Keyboard Support (Autodesk Fusion 360 design; units mm, degrees)
Autodesk Fusion 360 part; units mm, degrees
sketch "Sketch1" plane through (0, 0, 0) normal (0, 0, 1) x (1, 0, 0)
  line L0 (0, 0) -> (280, 0)
  line L1 (280, 0) -> (280, 6)
  line L2 (280, 6) -> (0, 6)
  line L3 (0, 6) -> (0, 0)
  line L4 (280, 6) -> (0, 6)
  line L5 (0, 6) -> (0, 26)
  line L6 (0, 26) -> (280, 26)
  line L7 (280, 26) -> (280, 6)
  line L8 (140, 26) -> (140, 66) construction
  line L9 (140, 66) -> (150, 66)
  line L10 (150, 66) -> (150, 26)
  line L11 (150, 26) -> (140, 26)
  line L12 (140, 26) -> (140, 66)
  line L13 (140, 66) -> (130, 66)
  line L14 (130, 66) -> (130, 26)
  line L15 (130, 26) -> (140, 26)
  line L16 (140, 26) -> (140, 66)
  dimension "d1" = 280
  dimension "d2" = 6
  dimension "d9" = 20
  dimension "d10" = 280
  dimension "d11" = 40
  dimension "d12" = 10
  dimension "d13" = 10
  constraint horizontal L0
  constraint vertical L1
  constraint horizontal L2
  constraint vertical L3
  constraint coincident L0.start L3.end
  constraint horizontal L4
  constraint vertical L5
  constraint horizontal L6
  constraint vertical L7
  constraint midpoint L6 L8.start
  constraint perpendicular L6 L8
  constraint horizontal L9
  constraint vertical L10
  constraint horizontal L11
  constraint vertical L12
  constraint horizontal L13
  constraint vertical L14
  constraint horizontal L15
  constraint vertical L16
  measures "d1" distance of L0.start L0.end
  measures "d2" distance of L0.start L2.end
  measures "d9" distance of L1.end L6.end
  measures "d10" distance of L5.end L6.end
  measures "d11" distance of L8.start L8.end
  measures "d12" distance of L8.end L9.end
  measures "d13" distance of L8.end L13.end
extrude "Extrude3" add sketch "Sketch1" along normal blind 4 contours L2 L4 L5 L6 L7 L11 L15 makes body 1
extrude "Extrude1" add sketch "Sketch1" along normal blind 10 separate body contours L0 L1 L2 L3 L4 makes body 2
extrude "Extrude4" add sketch "Sketch1" along normal blind 4 contours L6 L12 L13 L14 L15 L16 | L6 L9 L10 L11 L12 L16 bodies 1
sketch "Sketch3" plane through (150, 0, 0) normal (1, 0, 0) x (0, 1, 0)
  line L0 (26, 0) -> (66, 0)
  line L1 (66, 0) -> (66, 4)
  line L2 (66, 4) -> (26, 4)
  line L3 (26, 4) -> (26, 0)
  line L4 (6.0067, 5.0364) -> (66, 1.8987)
  constraint coincident L1 L4.end
extrude "Extrude5" cut sketch "Sketch3" against normal blind 20 contours L1 L2 L3 L4 bodies 1
sketch "Sketch4" plane through (0, 0, 0) normal (0, 0, 1) x (1, 0, 0)
  line L0 (0, -45.217) -> (280, -45.217)
  line L1 (280, -45.217) -> (280, -50.217)
  line L2 (280, -50.217) -> (0, -50.217)
  line L3 (0, -50.217) -> (0, -45.217)
  dimension "d20" = 280
  dimension "d21" = 5
  constraint horizontal L0
  constraint vertical L1
  constraint horizontal L2
  constraint vertical L3
  measures "d20" distance of L0.start L0.end
  measures "d21" distance of L0.start L2.end
extrude "Extrude6" add sketch "Sketch4" along normal blind 5 separate body makes body 3
sketch "Sketch5" plane through (280, 0, 0) normal (1, 0, 0) x (0, 1, 0)
  line L0 (-50.217, 0) -> (-45.217, 0)
  line L1 (-45.217, 0) -> (-45.217, 5)
  line L2 (-45.217, 5) -> (-50.217, 5)
  line L3 (-50.217, 5) -> (-50.217, 0)
  line L4 (-45.217, 5) -> (-50.217, 0)
  constraint coincident L1.end L2.start
  constraint coincident L0.start L3.end
extrude "Extrude7" cut sketch "Sketch5" against normal blind 280 contours L2 L3 L4 bodies 3
fillet "Fillet1" radius 10 2 edges at (130, 66, 0.9493) (150, 66, 0.9493) on bodies 1
fillet "Fillet2" radius 10 1 edges at (280, 26, 2) on bodies 1
fillet "Fillet3" radius 10 1 edges at (0, 26, 2) on bodies 1
combine "Combine1" operation add target body 1 tool bodies 2
